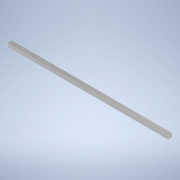
# Autodesk Inventor part: ロボットベース15x15_3
Saved by Autodesk Inventor 2020.3 (Build 243373000, 373)
## iProperties
Created: 2020-07-04
Part Number: ロボットベース15x15_3
Material: アルミニウム 6061
Document SubType Name: Modeling
Designer: totot
Density: 2.7 g/cm^3
Appearance: アルミニウム - フラット
Mass: 115.336 g
Surface Area: 727.072 cm^2
Volume: 42.7169 cm^3
Author: totot
Autodesk Inventor part; units mm, degrees
ref_plane "YZ Plane" through (0, 0, 0) normal (1, 0, 0) x (0, 1, 0)
ref_plane "XZ Plane" through (0, 0, 0) normal (0, 1, 0) x (-1, 0, 0)
ref_plane "XY Plane" through (0, 0, 0) normal (0, 0, 1) x (1, 0, 0)
sketch "スケッチ1" plane through (0, 0, 0) normal (1, 0, 0) x (0, 1, 0)
  line L0 (0, 0) -> (-15, 0)
  line L1 (-15, 0) -> (-15, 15)
  line L2 (-15, 15) -> (0, 15)
  line L3 (0, 15) -> (0, 0)
  line L4 (-1.2, 13.8) -> (-13.8, 13.8)
  line L5 (-13.8, 13.8) -> (-13.8, 1.2)
  line L6 (-13.8, 1.2) -> (-1.2, 1.2)
  line L7 (-1.2, 1.2) -> (-1.2, 13.8)
  dimension "d0" = 15
  dimension "d1" = 15
  dimension "d2" = 1.2
  dimension "d3" = 1.2
  dimension "d4" = 1.2
  dimension "d5" = 1.2
  constraints: 16 end point, 4 parallel, 2 horizontal, 2 perpendicular
  measures "d0" distance of L1.end L2.end
  measures "d1" distance of L0.end L1.end
  measures "d2" distance between parallel lines of L2 L4
  measures "d3" distance between parallel lines of L7 L3
  measures "d4" distance between parallel lines of L1 L5
  measures "d5" distance between parallel lines of L0 L6
extrude "押し出し1" add sketch "スケッチ1" along normal blind 116
sketch "スケッチ2" plane through (0, -15, 15) normal (0, 0, 1) x (1, 0, 0)
  line L0 (0, 15) -> (116, 15) projected
  line L1 (0, 15) -> (0, 0) projected
  line L2 (116, 15) -> (116, 0) projected
  point P0 (7.5, 7.5)
  point P1 (108.5, 7.5)
  dimension "d8" = 7.5
  dimension "d9" = 7.5
  dimension "d10" = 7.5
  dimension "d11" = 7.5
  measures "d8" distance from line of L0 point (7.5, 7.5)
  measures "d9" distance from line of point (108.5, 7.5) L0
  measures "d10" distance from line of point (7.5, 7.5) L1
  measures "d11" distance from line of point (108.5, 7.5) L2
hole "穴1" at (7.5, -7.5, 15) at (108.5, -7.5, 15) direction (0, 0, -1) diameter 3 end through all
sketch "スケッチ3" plane through (0, -15, 0) normal (0, 0, -1) x (-1, 0, 0)
  circle A0 centre (-7.5, 7.5) radius 1.5 projected
  line L0 (0, 0) -> (-116, 0) projected
  point P0 (0, 15)
  point P1 (-58, 7.5)
  dimension "d19" = 50.5
  dimension "d20" = 7.5
  measures "d19" distance of point (-58, 7.5) A0.centre
  measures "d20" distance from line of point (-58, 7.5) L0
hole "穴2" at (58, -7.5, 0) direction (0, 0, 1) diameter 5 end through all
sketch "スケッチ4" plane through (0, -15, 0) normal (0, -1, 0) x (1, 0, 0)
  line L0 (0, 15) -> (0, 0) projected
  line L1 (0, 0) -> (116, 0) projected
  line L2 (116, 15) -> (116, 0) projected
  point P0 (22.5, 7.5)
  point P1 (93.5, 7.5)
  dimension "d28" = 22.5
  dimension "d29" = 7.5
  dimension "d30" = 7.5
  dimension "d31" = 22.5
  measures "d28" distance from line of point (22.5, 7.5) L0
  measures "d29" distance from line of point (22.5, 7.5) L1
  measures "d30" distance from line of L1 point (93.5, 7.5)
  measures "d31" distance from line of point (93.5, 7.5) L2
hole "穴3" at (22.5, -15, 7.5) at (93.5, -15, 7.5) direction (0, 1, 0) diameter 3 end through all
sketch "スケッチ5" plane through (116, 0, 0) normal (1, 0, 0) x (0, 0, -1)
  line L0 (0, 0) -> (-15, 0)
  line L1 (-15, 0) -> (-15, -15)
  line L2 (-15, -15) -> (0, -15)
  line L3 (0, -15) -> (0, 0)
  line L4 (-13.8, -1.2) -> (-1.2, -1.2) projected
  line L5 (-1.2, -1.2) -> (-13.8, -1.2)
  line L6 (-13.8, -1.2) -> (-13.8, -13.8)
  line L7 (-13.8, -13.8) -> (-1.2, -13.8)
  line L8 (-1.2, -13.8) -> (-1.2, -1.2)
  dimension "d39" = 15
  dimension "d40" = 15
  constraints: 16 end point, 4 parallel, 2 horizontal, 2 perpendicular
  measures "d39" distance of L2.end L1.end
  measures "d40" distance of L1.end L0.end
extrude "押し出し2" add sketch "スケッチ5" along normal blind 99
sketch "スケッチ6" plane through (0, -15, 0) normal (0, 0, -1) x (-1, 0, 0)
  line L0 (-215, 0) -> (-215, 15) projected
  line L1 (0, 15) -> (-215, 15) projected
  point P0 (-207.5, 7.5)
  dimension "d43" = 7.5
  dimension "d44" = 7.5
  measures "d43" distance from line of L0 point (-207.5, 7.5)
  measures "d44" distance from line of L1 point (-207.5, 7.5)
hole "穴4" at (207.5, -7.5, 0) direction (0, 0, 1) diameter 3 end through all
sketch "スケッチ7" plane through (0, 0, 15) normal (0, 1, 0) x (1, 0, 0)
  line L0 (0, 15) -> (215, 15) projected
  line L1 (215, 15) -> (215, 0) projected
  point P0 (192.5, 7.5)
  dimension "d52" = 7.5
  dimension "d53" = 22.5
  measures "d52" distance from line of L0 point (192.5, 7.5)
  measures "d53" distance from line of L1 point (192.5, 7.5)
hole "穴5" at (192.5, 0, 7.5) direction (0, -1, 0) diameter 3 end through all
sketch "スケッチ8" plane through (0, -15, 0) normal (0, 0, -1) x (-1, 0, 0)
  circle A0 centre (-108.5, 7.5) radius 1.5 projected
  line L0 (0, 0) -> (-215, 0) projected
  line L1 (-215, 0) -> (-215, 15) projected
  point P0 (0, 15)
  point P1 (-131, 7.5)
  point P2 (-177.5, 7.5)
  dimension "d61" = 22.5
  dimension "d62" = 7.5
  dimension "d63" = 7.5
  dimension "d64" = 37.5
  measures "d61" distance of point (-131, 7.5) A0.centre
  measures "d62" distance from line of point (-131, 7.5) L0
  measures "d63" distance from line of L0 point (-177.5, 7.5)
  measures "d64" distance from line of L1 point (-177.5, 7.5)
hole "穴6" at (131, -7.5, 0) at (177.5, -7.5, 0) direction (0, 0, 1) diameter 3 end through all
sketch "スケッチ9" plane through (0, 0, 15) normal (0, 1, 0) x (1, 0, 0)
  line L0 (0, 15) -> (215, 15) projected
  line L1 (0, 15) -> (0, 0) projected
  circle A0 centre (22.5, 7.5) radius 1.5 projected
  circle A1 centre (192.5, 7.5) radius 1.5 projected
  line L2 (215, 15) -> (215, 0) projected
  point P0 (5.625, 7.5)
  point P1 (11.25, 7.5)
  point P2 (209.375, 7.5)
  point P3 (203.75, 7.5)
  point P4 (187.5, 7.5)
  point P5 (27.5, 7.5)
  point P6 (16.875, 7.5)
  point P7 (198.125, 7.5)
  point P8 (32.5, 7.5)
  point P9 (37.5, 7.5)
  point P10 (42.5, 7.5)
  point P11 (47.5, 7.5)
  point P12 (52.5, 7.5)
  point P13 (57.5, 7.5)
  point P14 (62.5, 7.5)
  point P15 (67.5, 7.5)
  point P16 (72.5, 7.5)
  point P17 (77.5, 7.5)
  point P18 (82.5, 7.5)
  point P19 (87.5, 7.5)
  point P20 (182.3, 7.5)
  point P21 (177.1, 7.5)
  point P22 (171.9, 7.5)
  point P23 (166.7, 7.5)
  point P24 (161.5, 7.5)
  point P25 (156.3, 7.5)
  point P26 (151.1, 7.5)
  point P27 (145.9, 7.5)
  point P28 (140.7, 7.5)
  point P29 (135.5, 7.5)
  point P30 (130.3, 7.5)
  point P31 (125.1, 7.5)
  point P32 (119.9, 7.5)
  point P33 (114.7, 7.5)
  point P34 (109.5, 7.5)
  point P35 (104.3, 7.5)
  point P36 (99.1, 7.5)
  dimension "d72" = 7.5
  dimension "d74" = 7.5
  dimension "d75" = 7.5
  dimension "d76" = 5
  dimension "d77" = 22.5
  dimension "d78" = 5.625
  dimension "d79" = 5.625
  dimension "d80" = 7.5
  dimension "d81" = 5.625
  dimension "d82" = 7.5
  dimension "d83" = 7.5
  dimension "d84" = 7.5
  dimension "d85" = 5
  dimension "d86" = 22.5
  dimension "d87" = 7.5
  dimension "d88" = 5.625
  dimension "d89" = 5.625
  dimension "d90" = 5.625
  dimension "d93" = 5
  dimension "d100" = 5.2
  constraints: 2 horizontal, 29 other
  measures "d72" distance from line of L0 point (5.625, 7.5)
  measures "d74" distance from line of L0 point (11.25, 7.5)
  measures "d75" distance from line of L0 point (27.5, 7.5)
  measures "d76" distance of point (27.5, 7.5) A0.centre
  measures "d77" distance from line of L1 A0.centre
  measures "d78" distance from line of point (5.625, 7.5) L1
  measures "d79" distance of point (11.25, 7.5) point (5.625, 7.5)
  measures "d80" distance from line of L0 point (16.875, 7.5)
  measures "d81" distance of point (16.875, 7.5) point (11.25, 7.5)
  measures "d82" distance from line of L0 point (209.375, 7.5)
  measures "d83" distance from line of L0 point (203.75, 7.5)
  measures "d84" distance from line of L0 point (187.5, 7.5)
  measures "d85" distance of A1.centre point (187.5, 7.5)
  measures "d86" distance from line of L2 A1.centre
  measures "d87" distance from line of L0 point (198.125, 7.5)
  measures "d88" distance of point (198.125, 7.5) A1.centre
  measures "d89" distance of point (203.75, 7.5) point (198.125, 7.5)
  measures "d90" distance of point (209.375, 7.5) point (203.75, 7.5)
  measures "d93" distance of point (27.5, 7.5) point (32.5, 7.5)
  measures "d100" distance of point (187.5, 7.5) point (182.3, 7.5)
hole "穴7" at (5.625, 0, 7.5) at (11.25, 0, 7.5) at (209.375, 0, 7.5) at (203.75, 0, 7.5) at (187.5, 0, 7.5) at (27.5, 0, 7.5) at (16.875, 0, 7.5) at (198.125, 0, 7.5) at (32.5, 0, 7.5) at (37.5, 0, 7.5) at (42.5, 0, 7.5) at (47.5, 0, 7.5) at (52.5, 0, 7.5) at (57.5, 0, 7.5) at (62.5, 0, 7.5) at (67.5, 0, 7.5) at (72.5, 0, 7.5) at (77.5, 0, 7.5) at (82.5, 0, 7.5) at (87.5, 0, 7.5) at (182.3, 0, 7.5) at (177.1, 0, 7.5) at (171.9, 0, 7.5) at (166.7, 0, 7.5) at (161.5, 0, 7.5) at (156.3, 0, 7.5) at (151.1, 0, 7.5) at (145.9, 0, 7.5) at (140.7, 0, 7.5) at (135.5, 0, 7.5) at (130.3, 0, 7.5) at (125.1, 0, 7.5) at (119.9, 0, 7.5) at (114.7, 0, 7.5) at (109.5, 0, 7.5) at (104.3, 0, 7.5) at (99.1, 0, 7.5) direction (0, -1, 0) diameter 4 end through all
sketch "スケッチ11" plane through (215, 0, 0) normal (1, 0, 0) x (0, 0, -1)
  line L0 (0, -15) -> (0, 0) projected
  line L1 (-15, 0) -> (-15, -15) projected
  line L2 (0, 0) -> (-15, 0)
  line L3 (-15, 0) -> (-15, -15)
  line L4 (-15, -15) -> (0, -15)
  line L5 (0, -15) -> (0, 0)
  line L6 (-1.2, -13.8) -> (-13.8, -13.8) projected
  line L7 (-1.2, -1.2) -> (-13.8, -1.2)
  line L8 (-13.8, -1.2) -> (-13.8, -13.8)
  line L9 (-13.8, -13.8) -> (-1.2, -13.8)
  line L10 (-1.2, -13.8) -> (-1.2, -1.2)
  constraints: 16 end point, 4 parallel, 2 horizontal, 2 perpendicular
extrude "押し出し3" add sketch "スケッチ11" along normal blind 450
sketch "スケッチ12" plane through (0, -15, 0) normal (0, 0, -1) x (-1, 0, 0)
  line L0 (0, 15) -> (-665, 15) projected
  line L1 (-665, 0) -> (-665, 15) projected
  point P0 (-660, 7.5)
  point P1 (-560, 7.5)
  dimension "d114" = 7.5
  dimension "d115" = 5
  dimension "d116" = 7.5
  dimension "d117" = 100
  measures "d114" distance from line of point (-560, 7.5) L0
  measures "d115" distance from line of point (-660, 7.5) L1
  measures "d116" distance from line of point (-660, 7.5) L0
  measures "d117" distance of point (-660, 7.5) point (-560, 7.5)
hole "穴8" at (660, -7.5, 0) at (560, -7.5, 0) direction (0, 0, 1) diameter 3 end through all
equation "\"d3\" = d2"
equation "\"d4\" = d2"
equation "\"d5\" = d3"
equation "\"d9\" = d8"
equation "\"d10\" = d8"
equation "\"d11\" = d9"
equation "\"d30\" = d29"
equation "\"d31\" = d28"
equation "\"d63\" = d62"
equation "\"d78\" = 0.25 * d77"
equation "\"d79\" = d78"
equation "\"d80\" = d74"
equation "\"d81\" = d79"
equation "\"d88\" = 0.25 * d86"
equation "\"d89\" = d88"
equation "\"d90\" = d89"
equation "\"d116\" = d114"
